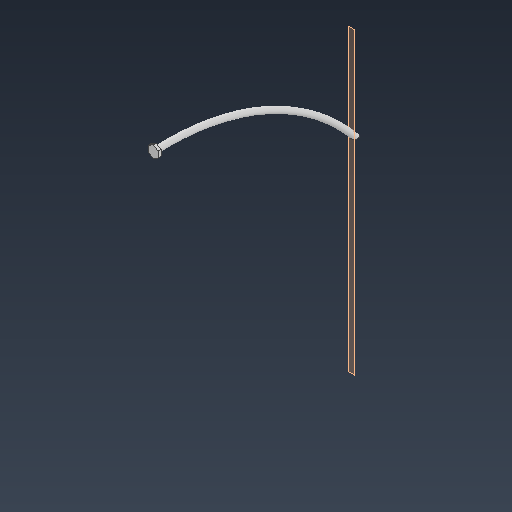
# Autodesk Inventor part: large_hoop
Saved by Autodesk Inventor 2021 (Build 250183000, 183)
## iProperties
Created: 2021-05-05
Part Number: large_hoop
Material: Generic
Document SubType Name: Modeling
Density: 1 g/cm^3
Appearance: Default
Autodesk Inventor part; units mm, degrees
ref_plane "YZ Plane" through (0, 0, 0) normal (1, 0, 0) x (0, 1, 0)
ref_plane "XZ Plane" through (0, 0, 0) normal (0, 1, 0) x (-1, 0, 0)
sketch "Sketch1" plane through (0, 0, 0) normal (1, 0, 0) x (0, 1, 0)
  circle A0 centre (0, 0) radius 1650
  dimension "d0" = 3300
  constraints: 1 centre point, 1 coincident
  measures "d0" diameter of A0
sketch "Sketch2" plane through (0, 0, 0) normal (0, 0, 1) x (1, 0, 0)
  circle A0 centre (0, 1650) radius 20
  point P0 (0, 0)
  dimension "d1" = 1650
  dimension "d2" = 0
  dimension "d3" = 40
  constraints: 1 centre point
  measures "d1" distance of A0.centre point (0, 0)
  measures "d2" horizontal distance of A0.centre point (0, 0)
  measures "d3" diameter of A0
sweep "Sweep1" add profiles "Sketch2" path "Sketch1"
sketch "Sketch3" plane through (0, 0, 0) normal (0, 0, 1) x (1, 0, 0)
  circle A0 centre (0, 1650) radius 15
  point P0 (0, 0)
  dimension "d6" = 30
  dimension "d7" = 0
  dimension "d8" = 1650
  constraints: 1 centre point
  measures "d6" diameter of A0
  measures "d7" horizontal distance of A0.centre point (0, 0)
  measures "d8" distance of point (0, 0) A0.centre
sweep "Sweep2" cut profiles "Sketch3" path "Sketch1"
sketch "Sketch4" plane through (0, 0, 0) normal (1, 0, 0) x (0, 1, 0)
  line L0 (1050, 1730) -> (1050, -1730)
  line L1 (1050, 80) -> (2780, 80)
  line L2 (2780, 80) -> (2780, 1730)
  line L3 (1050, 1730) -> (1180.0646, 1730)
  line L4 (1180.0646, 1730) -> (2780, 1730)
  line L5 (1050, 1730) -> (-1730, 1730)
  line L6 (-1730, 1730) -> (-1730, -1730)
  line L7 (-1730, -1730) -> (1050, -1730)
  point P0 (0, 0)
  dimension "d12" = 3460
  dimension "d13" = 1730
  dimension "d14" = 1050
  dimension "d15" = 1730
  dimension "d16" = 1730
  dimension "d17" = 80
  constraints: 17 end point, 2 horizontal, 2 perpendicular, 2 point on line, 2 vertical
  measures "d12" distance of L0.start L0.end
  measures "d13" vertical distance of point (0, 0) L0.start
  measures "d14" distance from line of point (0, 0) L0
  measures "d15" distance from line of point (0, 0) L6
  measures "d16" distance of L1.start L1.end
  measures "d17" distance from line of point (0, 0) L1
extrude "Extrusion1" cut sketch "Sketch4" along normal mid plane 80
sketch "Sketch5" plane through (0, 1050, -1272.6852) normal (0, -1, 0) x (1, 0, 0)
  line L0 (2.5, -4.2386) -> (-2.5, -4.2386)
  line L1 (-2.5, -4.2386) -> (-2.5, 41.1701)
  line L2 (-2.5, 41.1701) -> (2.5, 41.1701)
  line L3 (2.5, 41.1701) -> (2.5, -4.2386)
  line L4 (0, 1628.4117) -> (0, -301.6563) projected
  point P0 (0, 1272.6852)
  dimension "d20" = 5
  dimension "d21" = 2.5
  constraints: 8 end point, 2 parallel, 1 horizontal, 1 perpendicular
  measures "d20" distance between parallel lines of L1 L3
  measures "d21" distance between parallel lines of L4 L1
extrude "Extrusion2" cut sketch "Sketch5" against normal blind 5
fillet "Fillet2" radius 2 2 edges at (0, 1055, -1249.0797) (0, 1055, -1242.5277)
ref_plane "Work Plane1" through (0, 0, -1250) normal (0, 0, 1) x (1, 0, 0)
sketch "Sketch6" plane through (0, 1648.0592, 80) normal (0, 0, 1) x (1, 0, 0)
  line L0 (0, 370.5272) -> (0, -1984.4902) projected
  line L1 (0, 40.4032) -> (-34.641, 20.4032)
  line L2 (-34.641, 20.4032) -> (-34.641, -19.5968)
  line L3 (-34.641, -19.5968) -> (0, -39.5968)
  line L4 (0, -39.5968) -> (34.641, -19.5968)
  line L5 (34.641, -19.5968) -> (34.641, 20.4032)
  line L6 (34.641, 20.4032) -> (0, 40.4032)
  point P0 (0, -1648.0592)
  dimension "d32" = 120
  dimension "d33" = 120
  dimension "d34" = 40
  dimension "d35" = 120
  dimension "d36" = 120
  dimension "d37" = 120
  constraints: 12 end point, 3 equal length, 1 point on line, 1 vertical
  measures "d32" angle of L1 L2
  measures "d33" angle of L2 L3
  measures "d34" distance of L1.end L2.end
  measures "d35" angle of L5 L4
  measures "d36" angle of L6 L5
  measures "d37" angle of L4 L3
extrude "Extrusion4" add sketch "Sketch6" along normal blind 20
equation "\"d0\" = hoop_radius_large"
equation "\"d1\" = 0.5 * d0"
equation "\"d3\" = hoop_width_small"
equation "\"d6\" = hoop_width_small - hoop_thickness_small"
equation "\"d8\" = 0.5 * d0"
equation "\"d12\" = 2 * hoop_width_large + d0"
equation "\"d13\" = 0.5 * d12"
equation "\"d14\" = 0.5 * hoop_radius_large - hoop_height_small"
equation "\"d15\" = 0.5 * d12"
equation "\"d16\" = d13"
equation "\"d17\" = hoop_width_large"
equation "\"d18\" = hoop_width_large"
equation "\"d20\" = hoop_cable_diam"
equation "\"d21\" = 0.5 * d20"
equation "\"d22\" = hoop_cable_diam"
equation "\"hoop_radius_large\" = 3300"
equation "\"hoop_width_large\" = 80"
equation "\"hoop_thickness_small\" = 10"
equation "\"hoop_width_small\" = 40"
equation "\"rack_tooth_thickness\" = 5"
equation "\"rack_tooth_addendum\" = 5"
equation "\"rack_tooth_dedendum\" = 5"
equation "\"hoop_bearing_length\" = 5deg"
equation "\"hoop_cable_diam\" = 5"
equation "\"secure_arm_radii\" = 9"
equation "\"secure_arm_hold_length\" = 35"
equation "\"secure_arm_angle\" = 20deg"
equation "\"hoop_cable_pulley_diam\" = 22"
equation "\"support_frame_squareBarThickness\" = 5"
equation "\"support_frame_squareBarFillet\" = 2"
equation "\"support_baseClamp_platformThickness\" = 15"
equation "\"support_baseClamp_platformWidthBuffer\" = 0"
equation "\"support_baseClamp_platformLengthBuffer\" = 35"
equation "\"support_frame_endHoleBuffer\" = 25"
equation "\"support_baseClamp_thickness\" = 8"
equation "\"support_baseClamp_sleeveSweepTerminationAngle\" = 55deg"
equation "\"support_baseClamp_sleeveHoleDiameter\" = 12"
equation "\"hoop_angle_z\" = 45deg"
equation "\"hoop_tabs_hole\" = 12"
equation "\"hoop_tabs_thickness\" = 6"
equation "\"wheelchair_deployed_length\" = 1067"
equation "\"wheelchair_deployed_height\" = 914"
equation "\"wheelchair_deployed_width\" = 635"
equation "\"sm_varx_member_tolerance\" = 0.5"
equation "\"sm_varx_squareBarThickness\" = 2.5"
equation "\"sm_varx_pinPlate_holeDiameter\" = 5"
equation "\"sm_varx_pinPlate_thickness\" = 5"
equation "\"hoop_height_small\" = 600"
body "Solid1"
